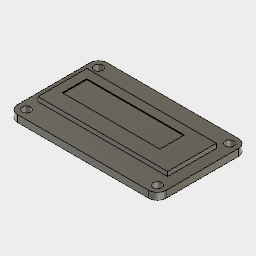
931 OLED 128x32 I2C (Autodesk Fusion 360 design; units mm, degrees)
Autodesk Fusion 360 part; units mm, degrees
sketch "Sketch1" plane through (0, 0, 0) normal (0, 0, 1) x (1, 0, 0)
  line L0 (0, 0) -> (34.036, 0)
  line L1 (34.036, 0) -> (34.036, 20.574)
  line L2 (34.036, 20.574) -> (0, 20.574)
  line L3 (0, 20.574) -> (0, 0)
  circle A0 centre (2, 18.574) radius 1
  line L4 (17.018, 20.574) -> (17.018, 0) construction
  line L5 (34.036, 10.287) -> (0, 10.287) construction
  circle A1 centre (32.036, 18.574) radius 1
  circle A2 centre (32.036, 2) radius 1
  circle A3 centre (2, 2) radius 1
  dimension "d1" = 34.036
  dimension "d2" = 20.574
  dimension "d3" = 2
  dimension "d5" = 2
  dimension "d23" = 2
  measures "d1" distance of L1.end L2.end
  measures "d2" distance of L0.end L1.end
  measures "d3" diameter of A0
  measures "d5" distance of L3 A0.centre
  measures "d23" distance of L2 A0.centre
extrude "Extrude1" add sketch "Sketch1" against normal blind 1.6
fillet "Fillet1" radius 2 4 edges at (0, 0, -0.8) (0, 20.574, -0.8) (34.036, 20.574, -0.8) (34.036, 0, -0.8)
sketch "Sketch2" plane through (0, 0, 0) normal (0, 0, 1) x (-1, 0, 0)
  arc A0 (-32.036, 0) -> (-34.036, -2) centre (-32.036, -2) ccw
  line L0 (-34.036, -2) -> (-34.036, -18.574)
  arc A1 (-34.036, -18.574) -> (-32.036, -20.574) centre (-32.036, -18.574) ccw
  line L1 (-32.036, -20.574) -> (-2, -20.574)
  arc A2 (-2, -20.574) -> (0, -18.574) centre (-2, -18.574) ccw
  line L2 (0, -18.574) -> (0, -2)
  arc A3 (0, -2) -> (-2, 0) centre (-2, -2) ccw
  line L3 (-2, 0) -> (-32.036, 0)
  circle A4 centre (-2, -2) radius 1
  circle A5 centre (-32.036, -18.574) radius 1
  circle A6 centre (-2, -18.574) radius 1
  circle A7 centre (-32.036, -2) radius 1
  line L4 (-1.778, -16.074) -> (-31.478, -16.074)
  line L5 (-31.478, -16.074) -> (-31.478, -4.898)
  line L6 (-31.478, -4.898) -> (-1.778, -4.898)
  line L7 (-1.778, -4.898) -> (-1.778, -16.074)
  dimension "d24" = 29.7
  dimension "d25" = 11.176
  dimension "d26" = 4.5
  dimension "d27" = 1.778
  measures "d24" distance of L4.start L4.end
  measures "d25" distance of L4.start L6.end
  measures "d26" distance of L1 L4
  measures "d27" distance of L2 L7
extrude "Extrude2" add sketch "Sketch2" along normal blind 1 contours L4 L5 L6 L7
sketch "Sketch3" plane through (0, 0, 1) normal (0, 0, 1) x (-1, 0, 0)
  line L0 (-1.778, -4.898) -> (-31.478, -4.898)
  line L1 (-31.478, -4.898) -> (-31.478, -16.074)
  line L2 (-31.478, -16.074) -> (-1.778, -16.074)
  line L3 (-1.778, -16.074) -> (-1.778, -4.898)
  line L4 (-3.81, -14.042) -> (-26.162, -14.042)
  line L5 (-26.162, -14.042) -> (-26.162, -8.454)
  line L6 (-26.162, -8.454) -> (-3.81, -8.454)
  line L7 (-3.81, -8.454) -> (-3.81, -14.042)
  dimension "d30" = 2.032
  dimension "d31" = 22.352
  dimension "d32" = 5.588
  dimension "d33" = 2.032
  measures "d30" distance of L3 L7
  measures "d31" distance of L4.start L4.end
  measures "d32" distance of L4.end L5.end
  measures "d33" distance of L2 L4
extrude "Extrude3" cut sketch "Sketch3" against normal blind 0.2 contours L4 L5 L6 L7
